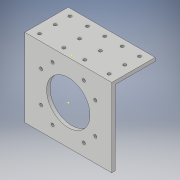
# Autodesk Inventor part: ousterholderm600
Saved by Autodesk Inventor 2019 (Build 230136000, 136)
## iProperties
Created: 2019-07-12
Part Number: ousterholderm600
Material: Generic
Document SubType Name: Modeling
Designer: Dell
Density: 1 g/cm^3
Appearance: Default
Author: Dell
Autodesk Inventor part; units mm, degrees
ref_plane "YZ Plane" through (0, 0, 0) normal (1, 0, 0) x (0, 1, 0)
ref_plane "XZ Plane" through (0, 0, 0) normal (0, 1, 0) x (-1, 0, 0)
ref_plane "XY Plane" through (0, 0, 0) normal (0, 0, 1) x (1, 0, 0)
sketch "Sketch3" plane through (0, 0, 0) normal (0, 0, 1) x (1, 0, 0)
  line L0 (-50, 45) -> (50, 45)
  line L1 (50, 45) -> (50, -45)
  line L2 (50, -45) -> (-50, -45)
  line L3 (-50, -45) -> (-50, 45)
  line L4 (-50, 45) -> (50, -45) construction
  line L5 (50, 45) -> (-50, -45) construction
  point P0 (0, 0)
  dimension "d4" = 100
  dimension "d5" = 90
  constraints: 12 end point, 2 midpoint, 2 parallel, 1 horizontal, 1 perpendicular
  measures "d4" distance of L1.end L2.end
  measures "d5" distance of L0.end L1.end
extrude "Extrusion2" add sketch "Sketch3" along normal blind 4
sketch "Sketch4" plane through (0, 0, 4) normal (0, 0, 1) x (1, 0, 0)
  point P0 (0, 0)
sketch "Sketch5" plane through (0, 0, 4) normal (0, 0, 1) x (1, 0, 0)
  line L0 (50, 45) -> (-50, 45) projected
  line L1 (50, 45) -> (-50, 45)
  line L2 (-50, 45) -> (-50, 41)
  line L3 (-50, 41) -> (50, 41)
  line L4 (50, 41) -> (50, 45)
  point P0 (0, 0)
  dimension "d8" = 4
  dimension "d9" = 100
  constraints: 8 end point, 2 parallel, 1 horizontal, 1 perpendicular
  measures "d8" distance of L1.end L2.end
  measures "d9" distance of L2.end L3.end
extrude "Extrusion3" add sketch "Sketch5" against normal blind 50
sketch "Sketch6" plane through (0, 0, 4) normal (0, 0, 1) x (1, 0, 0)
  line L0 (18, -31.18) -> (-18, -31.18)
  line L1 (-18, -31.18) -> (-18, 31.18)
  line L2 (-18, 31.18) -> (18, 31.18)
  line L3 (18, 31.18) -> (18, -31.18)
  line L4 (18, -31.18) -> (-18, 31.18) construction
  line L5 (-18, -31.18) -> (18, 31.18) construction
  circle A0 centre (-18, 31.18) radius 1.75
  circle A1 centre (18, 31.18) radius 1.75
  circle A2 centre (-18, -31.18) radius 1.75
  circle A3 centre (18, -31.18) radius 1.75
  point P0 (0, 0)
  dimension "d12" = 36
  dimension "d13" = 62.36
  dimension "d14" = 3.5
  dimension "d15" = 3.5
  dimension "d16" = 3.5
  dimension "d17" = 3.5
  constraints: 12 end point, 4 centre point, 4 coincident, 2 midpoint, 2 parallel, 1 horizontal, 1 perpendicular
  measures "d12" distance of L1.end L2.end
  measures "d13" distance of L0.end L1.end
  measures "d14" diameter of A0
  measures "d15" diameter of A1
  measures "d16" diameter of A2
  measures "d17" diameter of A3
extrude "Extrusion4" cut sketch "Sketch6" against normal blind 50 contours A2 L1 L0 | L0 L1 A2 | A3 L3 L0 | L0 L3 A3 | A0 L2 L1 | L1 L2 A0 | A1 L2 L3 | L3 L2 A1
sketch "Sketch7" plane through (0, 0, 4) normal (0, 0, 1) x (1, 0, 0)
  line L0 (31.18, -18) -> (-31.18, -18)
  line L1 (-31.18, -18) -> (-31.18, 18)
  line L2 (-31.18, 18) -> (31.18, 18)
  line L3 (31.18, 18) -> (31.18, -18)
  line L4 (31.18, -18) -> (-31.18, 18) construction
  line L5 (-31.18, -18) -> (31.18, 18) construction
  circle A0 centre (-31.18, 18) radius 1.75
  circle A1 centre (31.18, 18) radius 1.75
  circle A2 centre (-31.18, -18) radius 1.75
  circle A3 centre (31.18, -18) radius 1.75
  point P0 (0, 0)
  dimension "d20" = 62.36
  dimension "d21" = 36
  dimension "d22" = 3.5
  dimension "d23" = 3.5
  dimension "d24" = 3.5
  dimension "d25" = 3.5
  constraints: 12 end point, 4 centre point, 4 coincident, 2 midpoint, 2 parallel, 1 horizontal, 1 perpendicular
  measures "d20" distance of L1.end L2.end
  measures "d21" distance of L0.end L1.end
  measures "d22" diameter of A0
  measures "d23" diameter of A1
  measures "d24" diameter of A2
  measures "d25" diameter of A3
extrude "Extrusion5" cut sketch "Sketch7" against normal blind 50 contours A2 L1 L0 | L0 L1 A2 | A3 L3 L0 | L0 L3 A3 | A0 L2 L1 | L1 L2 A0 | A1 L2 L3 | L3 L2 A1
sketch "Sketch8" plane through (0, 0, 4) normal (0, 0, 1) x (1, 0, 0)
  circle A0 centre (0, 0) radius 25
  dimension "d28" = 50
  constraints: 1 centre point, 1 coincident
  measures "d28" diameter of A0
extrude "Extrusion6" cut sketch "Sketch8" against normal blind 43.6625
sketch "Sketch9" plane through (-50, 45, 4) normal (0, 1, 0) x (1, 0, 0)
  line L0 (0, 50) -> (0, 0) projected
  line L1 (100, 0) -> (0, 0) projected
  line L2 (0, 0) -> (38, 0)
  line L3 (38, 0) -> (38, 7)
  line L4 (38, 7) -> (0, 7)
  line L5 (0, 7) -> (0, 0)
  circle A0 centre (38, 7) radius 1.75
  line L6 (0, 0) -> (38, 0)
  line L7 (38, 0) -> (38, 25)
  line L8 (38, 25) -> (0, 25)
  line L9 (0, 25) -> (0, 0)
  circle A1 centre (38, 25) radius 1.75
  point P0 (50, 4)
  dimension "d31" = 38
  dimension "d32" = 7
  dimension "d36" = 3.5
  dimension "d39" = 25
  dimension "d40" = 3.5
  constraints: 16 end point, 5 equal length, 2 centre point, 2 coincident, 2 perpendicular, 1 point on line
  measures "d31" distance of L3.end L4.end
  measures "d32" distance of L2.end L3.end
  measures "d36" diameter of A0
  measures "d39" distance of L7.end L2.end
  measures "d40" diameter of A1
sketch "Sketch10" plane through (-50, 45, 4) normal (0, 1, 0) x (1, 0, 0)
  line L0 (100, 4) -> (100, 0) projected
  line L1 (100, 0) -> (0, 0) projected
  line L2 (100, 0) -> (62, 0)
  line L3 (62, 0) -> (62, 7)
  line L4 (62, 7) -> (100, 7)
  line L5 (100, 7) -> (100, 0)
  circle A0 centre (62, 7) radius 1.75
  line L6 (100, 0) -> (62, 0)
  line L7 (62, 0) -> (62, 25)
  line L8 (62, 25) -> (100, 25)
  line L9 (100, 25) -> (100, 0)
  line L10 (75, 0) -> (25, 0) projected
  circle A1 centre (62, 25) radius 1.75
  point P0 (50, 4)
  dimension "d33" = 38
  dimension "d34" = 7
  dimension "d35" = 3.5
  dimension "d37" = 25
  dimension "d38" = 3.5
  constraints: 16 end point, 4 parallel, 2 centre point, 2 coincident, 2 perpendicular, 1 collinear, 1 point on line
  measures "d33" distance of L0.end L2.end
  measures "d34" distance of L2.end L3.end
  measures "d35" diameter of A0
  measures "d37" distance of L2.end L7.end
  measures "d38" diameter of A1
sketch "Sketch11" plane through (-50, 45, 4) normal (0, 1, 0) x (1, 0, 0)
  point P0 (50, 4)
extrude "Extrusion7" cut sketch "Sketch9" against normal blind 43.6625 contours A1 L7 L8 | L8 L7 A1 | A0 L7 L4 | L4 L3 A0 | L7 A0 L3
extrude "Extrusion8" cut sketch "Sketch10" against normal blind 43.6625 contours A0 L3 L4 | L4 L7 A0 | L3 A0 L7 | A1 L7 L8 | L8 L7 A1
sketch "Sketch12" plane through (-50, 45, 4) normal (0, 1, 0) x (1, 0, 0)
  line L0 (0, 0) -> (100, 0) projected
  line L1 (0, 0) -> (10, 0)
  line L2 (10, 0) -> (10, 7)
  line L3 (10, 7) -> (0, 7)
  line L4 (0, 7) -> (0, 0)
  line L5 (100, 0) -> (0, 0) projected
  line L6 (0, 0) -> (10, 0)
  line L7 (10, 0) -> (10, 25)
  line L8 (10, 25) -> (0, 25)
  line L9 (0, 25) -> (0, 0)
  circle A0 centre (10, 7) radius 1.75
  circle A1 centre (10, 25) radius 1.75
  point P0 (50, 4)
  dimension "d45" = 10
  dimension "d46" = 7
  dimension "d47" = 25
  dimension "d48" = 3.5
  dimension "d49" = 3.5
  constraints: 16 end point, 4 parallel, 2 centre point, 2 coincident, 2 perpendicular, 1 collinear, 1 point on line
  measures "d45" distance of L0.start L1.end
  measures "d46" distance of L2.end L1.end
  measures "d47" distance of L7.end L1.end
  measures "d48" diameter of A0
  measures "d49" diameter of A1
extrude "Extrusion9" cut sketch "Sketch12" against normal blind 43.6625 contours A0 L3 L2 | L2 L7 A0 | A0 L7 L3 | A1 L7 L8 | L8 L7 A1
sketch "Sketch13" plane through (-50, 45, 4) normal (0, 1, 0) x (1, 0, 0)
  line L0 (0, 0) -> (100, 0) projected
  line L1 (100, 0) -> (90, 0)
  line L2 (90, 0) -> (90, 7)
  line L3 (90, 7) -> (100, 7)
  line L4 (100, 7) -> (100, 0)
  line L5 (100, 0) -> (90, 0)
  line L6 (90, 0) -> (90, 25)
  line L7 (90, 25) -> (100, 25)
  line L8 (100, 25) -> (100, 0)
  circle A0 centre (90, 25) radius 1.75
  circle A1 centre (90, 7) radius 1.75
  point P0 (50, 4)
  dimension "d52" = 10
  dimension "d53" = 7
  dimension "d54" = 25
  dimension "d55" = 3.5
  dimension "d56" = 3.5
  constraints: 16 end point, 4 parallel, 2 centre point, 2 coincident, 2 perpendicular, 1 collinear, 1 point on line
  measures "d52" distance of L0.end L1.end
  measures "d53" distance of L1.end L2.end
  measures "d54" distance of L1.end L6.end
  measures "d55" diameter of A0
  measures "d56" diameter of A1
extrude "Extrusion10" cut sketch "Sketch13" against normal blind 43.6625 contours A1 L6 L2 | L2 L3 A1 | L6 A1 L3 | A0 L7 L6 | L6 L7 A0
sketch "Sketch14" plane through (-50, 45, 4) normal (0, 1, 0) x (1, 0, 0)
  point P0 (50, 4)
sketch "Sketch15" plane through (-50, 45, 4) normal (0, 1, 0) x (1, 0, 0)
  line L0 (0, 50) -> (100, 50) projected
  line L1 (0, 50) -> (50, 50)
  line L2 (50, 50) -> (50, 42)
  line L3 (50, 42) -> (0, 42)
  line L4 (0, 42) -> (0, 50)
  line L5 (0, 50) -> (10, 50)
  line L6 (10, 50) -> (10, 42)
  line L7 (10, 42) -> (0, 42)
  line L8 (0, 42) -> (0, 50)
  line L9 (0, 4) -> (0, 50) projected
  line L10 (0, 50) -> (30, 50)
  line L11 (30, 50) -> (30, 42)
  line L12 (30, 42) -> (0, 42)
  line L13 (0, 42) -> (0, 50)
  line L14 (100, 4) -> (100, 50) projected
  line L15 (100, 50) -> (90, 50)
  line L16 (90, 50) -> (90, 42)
  line L17 (90, 42) -> (100, 42)
  line L18 (100, 42) -> (100, 50)
  line L19 (100, 50) -> (0, 50) projected
  line L20 (100, 50) -> (70, 50)
  line L21 (70, 50) -> (70, 42)
  line L22 (70, 42) -> (100, 42)
  line L23 (100, 42) -> (100, 50)
  circle A0 centre (50, 42) radius 1.75
  circle A1 centre (30, 42) radius 1.75
  circle A2 centre (10, 42) radius 1.75
  circle A3 centre (70, 42) radius 1.75
  circle A4 centre (90, 42) radius 1.75
  point P0 (50, 4)
  dimension "d59" = 50
  dimension "d60" = 8
  dimension "d61" = 10
  dimension "d62" = 30
  dimension "d63" = 10
  dimension "d64" = 30
  dimension "d65" = 3.5
  dimension "d66" = 3.5
  dimension "d67" = 3.5
  dimension "d68" = 3.5
  dimension "d69" = 3.5
  constraints: 40 end point, 10 parallel, 5 centre point, 5 coincident, 5 perpendicular, 4 point on line, 1 midpoint
  measures "d59" distance of L0.start L1.end
  measures "d60" distance of L1.end L2.end
  measures "d61" distance of L0.start L5.end
  measures "d62" distance of L0.start L10.end
  measures "d63" distance of L0.end L15.end
  measures "d64" distance of L0.end L20.end
  measures "d65" diameter of A0
  measures "d66" diameter of A1
  measures "d67" diameter of A2
  measures "d68" diameter of A3
  measures "d69" diameter of A4
extrude "Extrusion11" cut sketch "Sketch15" against normal blind 43.6625 contours A2 L3 L6 | L6 L3 A2 | L3 A2 | A1 L3 L11 | L11 L3 A1 | A0 L3 L2 | L2 L3 A0 | L3 A1 | A3 L22 L21 | L21 L22 A3 | A4 L17 L16 | L16 L22 A4 | L17 A4 L22
body "Solid2"
